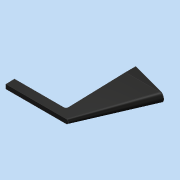
# Autodesk Inventor part: DivePlanesStabilizingFins
Saved by Autodesk Inventor 2017 (Build 210142000, 142)
## iProperties
Created: 2016-10-10
Part Number: DivePlanesStabilizingFins
Material: Generic
Document SubType Name: Modeling
Designer: techn
Density: 1 g/cm^3
Appearance: Glossy - Black
Author: techn
Autodesk Inventor part; units mm, degrees
ref_plane "YZ Plane" through (0, 0, 0) normal (1, 0, 0) x (0, 1, 0)
ref_plane "XZ Plane" through (0, 0, 0) normal (0, 1, 0) x (-1, 0, 0)
sketch "Sketch2" plane through (0, 0, 0) normal (0, 0, 1) x (1, 0, 0)
  line L0 (0, 0) -> (25.4, 0)
  line L1 (25.4, 0) -> (25.4, 6.35)
  line L2 (25.4, 6.35) -> (0, 6.35)
  line L3 (0, 6.35) -> (0, 0)
  arc A0 (25.4, 0) -> (25.4, 6.35) centre (25.4, 3.175) ccw
  dimension "d0" = 25.4
  dimension "d1" = 6.35
  constraints: 8 end point, 2 parallel, 2 point on circle, 2 tangent, 1 centre point, 1 horizontal, 1 perpendicular
  measures "d0" distance of L2.end L1.end
  measures "d1" distance of L1.end L0.end
ref_plane "Work Plane1" through (0, 0, 50.8) normal (0, 0, 1) x (1, 0, 0)
sketch "Sketch3" plane through (0, 0, 50.8) normal (0, 0, 1) x (1, 0, 0)
  line L0 (0, 1.5875) -> (6.35, 1.5875)
  line L1 (6.35, 1.5875) -> (6.35, 4.7625)
  line L2 (6.35, 4.7625) -> (0, 4.7625)
  line L3 (0, 4.7625) -> (0, 1.5875)
  arc A0 (6.35, 1.5875) -> (6.35, 4.7625) centre (6.35, 3.175) ccw
  point P0 (0, 0)
  dimension "d3" = 6.35
  dimension "d4" = 3.175
  dimension "d5" = 1.5875
  constraints: 8 end point, 2 parallel, 2 point on circle, 2 tangent, 1 centre point, 1 horizontal, 1 perpendicular
  measures "d3" distance of L2.end L1.end
  measures "d4" distance of L1.end L0.end
  measures "d5" distance of L0.start point (0, 0)
loft "Loft1" add profiles "Sketch2", "Sketch3"
sketch "Sketch4" plane through (0, 0, 0) normal (-1, 0, 0) x (0, 0, 1)
  line L0 (0, 6.35) -> (0, 0)
  line L1 (0, 0) -> (50.8, 1.5875)
  line L2 (50.8, 4.7625) -> (50.8, 1.5875)
  line L3 (0, 6.35) -> (50.8, 4.7625)
  line L4 (0, 6.35) -> (50.8, 4.7625)
  line L5 (44.45, 4.960938) -> (44.45, 1.389063)
  line L6 (50.8, 1.5875) -> (0, 0)
  dimension "d10" = 6.35
  constraints: 2 end point, 2 point on line, 1 vertical
  measures "d10" distance between parallel lines of L2 L5
extrude "Extrusion1" add sketch "Sketch4" along normal blind 38.608 contours L3 L2 L1 L5
sketch "Sketch5" plane through (25.4, 6.35, 0) normal (0, 0, -1) x (-1, 0, 0)
  line L0 (25.4, 0) -> (25.4, -6.35)
  line L1 (0, 0) -> (25.4, 0)
  arc A0 (0, 0) -> (0, -6.35) centre (0, -3.175) ccw
  line L2 (25.4, -6.35) -> (0, -6.35)
  line L3 (25.4, 0) -> (25.4, -6.35)
  line L4 (25.4, 0) -> (36.148692, 0)
  line L5 (36.148692, 0) -> (36.148692, -6.35)
  line L6 (36.148692, -6.35) -> (25.4, -6.35)
  line L7 (25.4, -6.35) -> (25.4, 0)
  line L8 (-3.175, -0.10761) -> (-3.175, -7.006989)
  constraints: 10 end point, 2 parallel, 1 horizontal, 1 perpendicular, 1 vertical
sketch "Sketch5 outline for Revolution1" plane through (25.4, 6.35, 0) normal (0, 0, -1) x (-1, 0, 0)
  line L0 (36.148692, 0) -> (0, 0)
  arc A0 (0, 0) -> (0, -6.35) centre (0, -3.175) ccw
  line L1 (0, -6.35) -> (36.148692, -6.35)
  line L2 (36.148692, -6.35) -> (36.148692, 0)
revolve "Revolution1" add sketch "Sketch5 outline for Revolution1" angle 15 about axis through (28.575, 6.24239, 0) along (0, -1, 0)
sketch "Sketch7" plane through (-10.748692, 6.35, 0) normal (0, 1, 0) x (1, 0, 0)
  line L0 (0, 0) -> (10.748692, 0)
  line L1 (36.148692, 0) -> (10.748692, 0)
  arc A0 (36.256878, 0.82175) -> (36.148692, 0) centre (39.323692, 0) ccw
  line L2 (1.339922, 10.17772) -> (36.256878, 0.82175)
  arc A1 (1.339922, 10.17772) -> (0, 0) centre (39.323692, 0) ccw
  line L3 (10.748692, 0) -> (10.748692, -44.45)
  line L4 (10.748692, 0) -> (-2.055619, 0)
  line L5 (-2.055619, 0) -> (-2.055619, 10.694673)
  line L6 (-2.055619, 10.694673) -> (10.748692, 10.694673)
  line L7 (10.748692, 10.694673) -> (10.748692, 0)
  constraints: 8 end point, 2 parallel, 1 horizontal, 1 perpendicular
extrude "Extrusion2" cut sketch "Sketch7" against normal blind 38.1 contours A1 L2 L7 L0 | L4 L5 L6 L7 L2 A1
fillet "Fillet1" radius 1.5875 1 edges at (0, 3.175, 44.45)
sketch "Sketch8" plane through (0, 0, -7.656648) normal (0.258819, 0, -0.9659258) x (-0.9659258, 0, -0.258819)
  line L0 (-29.583017, 3.175) -> (-24.820517, 3.175)
  line L1 (-24.820517, 3.175) -> (-8.945517, 3.175)
  circle A0 centre (-24.820517, 3.175) radius 1.397
  circle A1 centre (-8.945517, 3.175) radius 1.397
  line L2 (-26.408017, 0) -> (0, 0)
  point P0 (-1.981686, 0)
  dimension "d17" = 4.7625
  dimension "d18" = 15.875
  dimension "d19" = 2.794
  dimension "d20" = 2.794
  dimension "d23" = 3.175
  constraints: 4 end point, 2 centre point, 2 coincident, 1 horizontal, 1 point on line
  measures "d17" distance of L0.start L0.end
  measures "d18" distance of L0.end L1.end
  measures "d19" diameter of A0
  measures "d20" diameter of A1
  measures "d23" distance between parallel lines of L2 L1
extrude "Extrusion4" cut sketch "Sketch8" against normal blind 12.7
body "Solid1"
